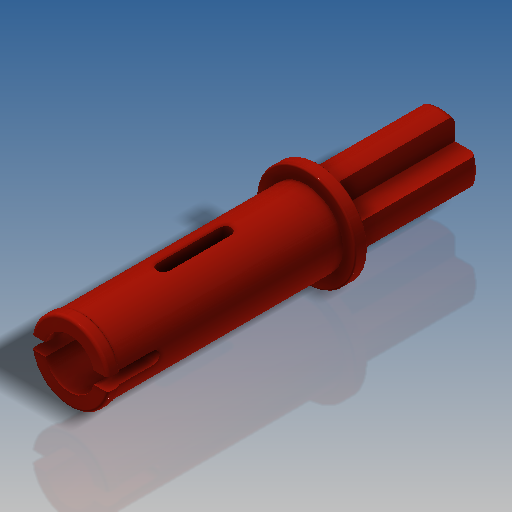
# Autodesk Inventor part: 11214-Red
Saved by Autodesk Inventor 2019.4 (Build 234330000, 330)
## iProperties
Created: 2014-06-03
Part Number: 11214-Red
Material: ABS Plastic
Document SubType Name: Modeling
Designer: D. Kohfeld
Appearance: Red
Density: 1.06 g/cm^3
Mass: 0.285147 g
Surface Area: 6.08598 cm^2
Volume: 0.269006 cm^3
Author: D. Kohfeld
Autodesk Inventor part; units mm, degrees
ref_plane "YZ Plane" through (0, 0, 0) normal (1, 0, 0) x (0, 1, 0)
ref_plane "XZ Plane" through (0, 0, 0) normal (0, 1, 0) x (-1, 0, 0)
ref_plane "XY Plane" through (0, 0, 0) normal (0, 0, 1) x (1, 0, 0)
sketch "Sketch1" plane through (0, 0, 0) normal (0, 1, 0) x (-1, 0, 0)
  line L0 (2.4, 15.2) -> (2.4, 0.8)
  line L1 (3.2, 0.8) -> (2.4, 0.8)
  line L2 (3.2, 0.8) -> (3.2, 0)
  line L3 (0, 0) -> (3.2, 0)
  line L4 (2.5, 16) -> (2.5, 15.2)
  line L5 (2.5, 16) -> (1.6, 16)
  line L6 (0, -3.2) -> (0, 19.2) projected
  line L7 (2.4, 15.2) -> (2.5, 15.2)
  line L8 (1.6, 16) -> (1.6, 0.8)
  line L9 (3.92, 0) -> (-1.12, 0) projected
  line L10 (-0.4, 10) -> (-0.4, 6)
  arc A0 (-0.4, 6) -> (0.4, 6) centre (0, 6) ccw
  line L11 (0.4, 6) -> (0.4, 10)
  arc A1 (0.4, 10) -> (-0.4, 10) centre (0, 10) ccw
  line L12 (1.6, 0.8) -> (0, 0.8)
  line L13 (0, 0.8) -> (0, 0)
  point P0 (2.4, 8)
  point P1 (0.4, 8)
  dimension "d1" = 4.8
  dimension "d2" = 5
  dimension "d6" = 16
  dimension "d7" = 0.8
  dimension "d8" = 6.4
  dimension "d9" = 0.8
  dimension "d16" = 4.8
  dimension "d17" = 0.8
  dimension "d31" = 3.2
  constraints: 24 end point, 4 point on circle, 4 point on line, 4 tangent, 3 perpendicular, 2 centre point, 2 horizontal alignment, 2 midpoint, 2 parallel, 1 horizontal
  measures "d1" diameter of L0 L6
  measures "d2" diameter of L4 L6
  measures "d6" distance between parallel lines of L5 L9
  measures "d7" distance from line of L4.end L5
  measures "d8" diameter of L2 L6
  measures "d9" distance between parallel lines of L1 L9
  measures "d17" diameter of A1
  measures "d31" diameter of L8 L6
revolve "Revolution1" add sketch "Sketch1" angle 360 about axis through (0, 0, -10) along (0, 0, 1) contours L0 L1 L2 L3 L6 L12 L8 L5 L4 L7
extrude "Extrusion1" cut sketch "Sketch1" along normal through all both and the other way through all contours A0 L10 A1 L6 | L6 A1 L11 A0
sketch "Sketch2" plane through (0, 0, 0) normal (1, 0, 0) x (0, 1, 0)
  line L0 (-1.6, 16) -> (1.6, 16) projected
  line L1 (-1.6, 0.8) -> (1.6, 0.8) projected
  line L2 (-0.4, 16) -> (0.4, 16)
  line L3 (0.4, 16) -> (0.4, 13)
  line L4 (-0.4, 13) -> (-0.4, 16)
  line L5 (0.4, 3.8) -> (0.4, 0.8)
  line L6 (0.4, 0.8) -> (-0.4, 0.8)
  line L7 (-0.4, 0.8) -> (-0.4, 3.8)
  arc A0 (-0.4, 13) -> (0.4, 13) centre (0, 13) ccw
  arc A1 (0.4, 3.8) -> (-0.4, 3.8) centre (0, 3.8) ccw
  point P0 (0, 0)
  point P1 (0, 16)
  point P2 (0, 16)
  point P3 (0, 0.8)
  point P4 (0, 0.8)
  dimension "d33" = 0.8
  dimension "d34" = 3.4
  constraints: 12 end point, 4 midpoint, 4 point on circle, 4 tangent, 2 centre point, 2 coincident, 2 horizontal, 2 parallel, 2 point on line, 1 collinear, 1 equal radius, 1 perpendicular, 1 vertical
  measures "d33" diameter of A0
extrude "Extrusion2" cut sketch "Sketch2" along normal through all both and the other way through all contours L0 L3 A0 L4
sketch "Sketch4" plane through (0, 0, 0) normal (0, 0, -1) x (-1, 0, 0)
  circle A0 centre (0, 0) radius 2.4 construction
  line L0 (-0.8, 2.2627) -> (-0.8, 0.8)
  line L1 (-0.8, 0.8) -> (-2.2627, 0.8)
  line L2 (-2.2627, -0.8) -> (-0.8, -0.8)
  line L3 (-0.8, -0.8) -> (-0.8, -2.2627)
  line L4 (0.8, -2.2627) -> (0.8, -0.8)
  line L5 (0.8, -0.8) -> (2.2627, -0.8)
  line L6 (2.2627, 0.8) -> (0.8, 0.8)
  line L7 (0.8, 0.8) -> (0.8, 2.2627)
  arc A1 (0.8, 2.2627) -> (-0.8, 2.2627) centre (0, 0) ccw
  arc A2 (-2.2627, 0.8) -> (-2.2627, -0.8) centre (0, 0) ccw
  arc A3 (-0.8, -2.2627) -> (0.8, -2.2627) centre (0, 0) ccw
  arc A4 (2.2627, -0.8) -> (2.2627, 0.8) centre (0, 0) ccw
  circle A5 centre (0, 0) radius 3.2 projected
  dimension "d39" = 4.8
  dimension "d40" = 1.6
  constraints: 16 end point, 8 point on circle, 7 equal length, 4 centre point, 4 perpendicular, 3 parallel, 1 coincident, 1 vertical, 14 other
  measures "d40" distance between parallel lines of L7 L0
extrude "Extrusion4" add sketch "Sketch4" along normal blind 8 contours A1 L7 L6 A4 L5 L4 A3 L3 L2 A2 L1 L0
fillet "Fillet1" radius 0.4 4 edges at (0, 2.4, -8) (2.4, 0, -8) (0, -2.4, -8) (-2.4, 0, -8)
fillet "Fillet1" radius 0.1 2 edges at (3.2, 0, 0.8) (3.2, 0, 0)
fillet "Fillet1" radius 0.2 4 edges at (0, 2.5, 16) (0, 2.5, 15.2) (0, -2.5, 16) (0, -2.5, 15.2)
equation "\"d1\" = tpd"
equation "\"d2\" = tpcd"
equation "\"d6\" = 2 * lu"
equation "\"d7\" = d9"
equation "\"d8\" = tsd"
equation "\"d9\" = tsl"
equation "\"d16\" = kd"
equation "\"d17\" = tpnw"
equation "\"d31\" = rd"
equation "\"d33\" = tpnw"
equation "\"d34\" = tpnl"
equation "\"d39\" = d41"
equation "\"d40\" = d42"
equation "\"d43\" = lu"
equation "\"d27\" = tf"
equation "\"d28\" = lf"
equation "\"d48\" = pinf"
equation "\"lf\" = 0.1"
equation "\"pinf\" = 0.2"
equation "\"tf\" = 0.4"
equation "\"tpd\" = 4.8"
equation "\"tpcd\" = 5"
equation "\"lu\" = 8"
equation "\"tsd\" = 6.4"
equation "\"tsl\" = 0.8"
equation "\"kd\" = 4.8"
equation "\"tpnw\" = 0.8"
equation "\"rd\" = 3.2"
equation "\"tpnl\" = 3.4"
equation "\"d41\" = 4.8"
equation "\"d42\" = 1.6"
body "Solid2"
